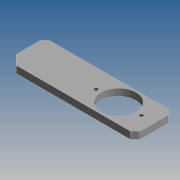
# Autodesk Inventor part: P126
Saved by Autodesk Inventor 2019 (Build 230136000, 136)
## iProperties
Created: 2017-01-30
Part Number: P126
Material: Aluminium
Document SubType Name: Modeling
Designer: serge.amoos
Density: 2.7 g/cm^3
Appearance: Par défaut
Description: Radiateur
Author: serge.amoos
Autodesk Inventor part; units mm, degrees
ref_plane "YZ Plane" through (0, 0, 0) normal (1, 0, 0) x (0, 1, 0)
ref_plane "XZ Plane" through (0, 0, 0) normal (0, 1, 0) x (-1, 0, 0)
ref_plane "XY Plane" through (0, 0, 0) normal (0, 0, 1) x (1, 0, 0)
sketch "Sketch1" plane through (0, 0, 0) normal (0, 0, 1) x (1, 0, 0)
  line L0 (-37.8, 0) -> (37.8, 0) projected
  line L1 (0, -11.2) -> (0, 11.2) projected
  line L2 (-27, 8) -> (27, 8)
  line L3 (27, 8) -> (27, -8)
  line L4 (27, -8) -> (-27, -8)
  line L5 (-27, -8) -> (-27, 8)
  point P0 (0, 0)
  point P1 (0, 8)
  point P2 (27, 0)
  dimension "d0" = 54
  dimension "d1" = 16
  constraints: 8 end point, 2 midpoint, 2 parallel, 2 point on line, 1 horizontal, 1 perpendicular
  measures "d0" distance of L2.start L2.end
  measures "d1" distance of L2.end L3.end
extrude "Extrusion1" add sketch "Sketch1" along normal blind 3
sketch "Sketch2" plane through (0, 0, 3) normal (0, 0, 1) x (1, 0, 0)
  line L0 (-37.8, 0) -> (37.8, 0) construction
  line L1 (0, -11.2) -> (0, 11.2) construction
  point P0 (0, 0)
  point P1 (12, 0)
  dimension "d4" = 12
  constraints: 1 point on line
  measures "d4" distance from line of point (12, 0) L1
hole "Hole1" at (12, 0, 3) direction (0, 0, -1) diameter 14.7 end through all
chamfer "Chamfer2" distance 2 angle 45 3 edges at (-27, 8, 1.5) (27, 8, 1.5) (27, -8, 1.5)
chamfer "Chamfer3" distance 4 angle 45 1 edges at (-27, -8, 1.5)
sketch "Sketch3" plane through (0, 0, 3) normal (0, 0, 1) x (1, 0, 0)
  line L0 (-37.8, 0) -> (37.8, 0) projected
  line L1 (0, -11.2) -> (0, 11.2) projected
  circle A0 centre (12, 0) radius 7.35 projected
  point P0 (0, 0)
  point P1 (2.47, 0)
  point P2 (21.53, 0)
  dimension "d21" = 9.53
  dimension "d22" = 9.53
  constraints: 2 point on line
  measures "d21" distance of A0.centre point (2.47, 0)
  measures "d22" distance of point (21.53, 0) A0.centre
hole "Hole2" at (2.47, 0, 3) at (21.53, 0, 3) direction (0, 0, -1) diameter 1.567 end through all thread size "M2x0.4" class "6H" standard "ISO Metric profile"
equation "\"d22\" = d21"
body "Solid1"
